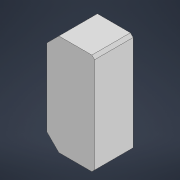
# Autodesk Inventor part: Carcasa
Saved by Autodesk Inventor 2022 (Build 260153000, 153)
## iProperties
Created: 2021-09-15
Part Number: Carcasa
Material: Generic
Document SubType Name: Sheet Metal
Designer: ARMU
Density: 1 g/cm^3
Sheet Metal Rule: Default
Appearance: Default
Author: ARMU
Autodesk Inventor part; units mm, degrees
ref_plane "YZ Plane" through (0, 0, 0) normal (1, 0, 0) x (0, 1, 0)
ref_plane "XZ Plane" through (0, 0, 0) normal (0, 1, 0) x (-1, 0, 0)
ref_plane "XY Plane" through (0, 0, 0) normal (0, 0, 1) x (1, 0, 0)
sketch "Sketch1" plane through (0, 0, 0) normal (0, 0, 1) x (1, 0, 0)
  line L0 (-272.7403, 778.9497) -> (12.2307, 778.9497)
  line L1 (12.2307, 778.9497) -> (35.7452, 755.4352)
  line L2 (35.7452, 755.4352) -> (35.7452, -69.5358)
  line L3 (35.7452, -69.5358) -> (12.2307, -93.0503)
  line L4 (12.2307, -93.0503) -> (-272.7403, -93.0503)
  line L5 (-376.2548, 10.4642) -> (-376.2548, 675.4352)
  line L6 (-376.2548, 675.4352) -> (-272.7403, 778.9497)
  line L7 (-376.2548, 10.4642) -> (-272.7403, -93.0503)
  circle A0 centre (35.7452, 778.9497) radius 23.5145 construction
  circle A1 centre (35.7452, -93.0503) radius 23.5145 construction
  circle A2 centre (-376.2548, 778.9497) radius 103.5145 construction
  circle A3 centre (-376.2548, -93.0503) radius 103.5145 construction
  line L8 (-271.4976, 775.9497) -> (-373.2548, 674.1926)
  line L9 (-373.2548, 674.1926) -> (-373.2548, 11.7068)
  line L10 (-373.2548, 11.7068) -> (-271.4976, -90.0503)
  line L11 (-271.4976, -90.0503) -> (10.9881, -90.0503)
  line L12 (10.9881, -90.0503) -> (32.7452, -68.2932)
  line L13 (32.7452, -68.2932) -> (32.7452, 754.1926)
  line L14 (32.7452, 754.1926) -> (10.9881, 775.9497)
  line L15 (10.9881, 775.9497) -> (-271.4976, 775.9497)
  line L16 (12.2307, -93.0503) -> (120.7988, -93.0503) construction
  line L17 (35.7452, -141.5714) -> (35.7452, 886.488) construction
  line L18 (124.1159, 778.9497) -> (-545.8501, 778.9497) construction
  line L19 (-376.2548, 913.6929) -> (-376.2548, -285.4862) construction
  line L20 (-520.4273, -93.0503) -> (301.4817, -93.0503) construction
  point P0 (0, 0)
  dimension "d2" = 47.029
  dimension "d0" = 872
  dimension "d1" = 412
  dimension "d3" = 47.029
  dimension "d4" = 207.029
  dimension "d5" = 207.029
  dimension "d6" = 3
  dimension "d7" = 3
  dimension "d8" = 3
  dimension "d9" = 3
  dimension "d10" = 3
  dimension "d11" = 3
  dimension "d12" = 3
  dimension "d13" = 3
  constraints: 42 end point, 12 point on line, 8 parallel, 6 point on circle, 4 vertical, 3 centre point, 3 horizontal, 2 collinear, 1 perpendicular, 1 vertical alignment, 2 other
  measures "d0" distance between parallel lines of L4 L0
  measures "d1" distance between parallel lines of L2 L5
  measures "d3" diameter of A1
  measures "d4" diameter of A2
  measures "d5" diameter of A3
  measures "d6" distance between parallel lines of L0 L15
  measures "d7" distance between parallel lines of L5 L9
  measures "d8" distance between parallel lines of L2 L13
  measures "d9" distance between parallel lines of L11 L4
  measures "d10" distance between parallel lines of L12 L3
  measures "d11" distance between parallel lines of L1 L14
  measures "d12" distance between parallel lines of L8 L6
  measures "d13" distance between parallel lines of L7 L10
extrude "Extrusion1" add sketch "Sketch1" along normal blind 330
sketch "Sketch2" plane through (0, 0, 330) normal (0, 0, 1) x (1, 0, 0)
  line L0 (-272.7403, 778.9497) -> (12.2307, 778.9497)
  line L1 (12.2307, 778.9497) -> (35.7452, 755.4352)
  line L2 (35.7452, 755.4352) -> (35.7452, -69.5358)
  line L3 (35.7452, -69.5358) -> (12.2307, -93.0503)
  line L4 (12.2307, -93.0503) -> (-272.7403, -93.0503)
  line L5 (-376.2548, 10.4642) -> (-376.2548, 675.4352)
  line L6 (-376.2548, 675.4352) -> (-272.7403, 778.9497)
  line L7 (-376.2548, 10.4642) -> (-272.7403, -93.0503)
  circle A0 centre (35.7452, 778.9497) radius 23.5145 construction
  circle A1 centre (35.7452, -93.0503) radius 23.5145 construction
  circle A2 centre (-376.2548, 778.9497) radius 103.5145 construction
  circle A3 centre (-376.2548, -93.0503) radius 103.5145 construction
  line L8 (12.2307, -93.0503) -> (120.7988, -93.0503) construction
  line L9 (35.7452, -141.5714) -> (35.7452, 886.488) construction
  line L10 (124.1159, 778.9497) -> (-545.8501, 778.9497) construction
  line L11 (-376.2548, 913.6929) -> (-376.2548, -285.4862) construction
  line L12 (-520.4273, -93.0503) -> (301.4817, -93.0503) construction
  point P0 (0, 0)
  point P1 (0, 0)
  dimension "d18" = 47.029
  dimension "d16" = 872
  dimension "d17" = 412
  dimension "d19" = 47.029
  dimension "d20" = 207.029
  dimension "d21" = 207.029
  constraints: 26 end point, 12 point on line, 6 point on circle, 4 vertical, 3 centre point, 3 horizontal, 2 collinear, 1 perpendicular, 1 vertical alignment, 2 other
  measures "d16" distance between parallel lines of L4 L0
  measures "d17" distance between parallel lines of L2 L5
  measures "d19" diameter of A1
  measures "d20" diameter of A2
  measures "d21" diameter of A3
extrude "Extrusion2" add sketch "Sketch2" along normal blind 3
equation "\"BendRadius\" = Thickness"
equation "\"BendReliefWidth\" = Thickness"
equation "\"BendReliefDepth\" = 0.5 * Thickness"
equation "\"CornerReliefSize\" = 4 * Thickness"
equation "\"MinimumRemnant\" = 2 * Thickness"
equation "\"TransitionRadius\" = BendRadius"
equation "\"JacobiRadiusSize\" = BendRadius"
equation "\"GapSize\" = Thickness"
equation "\"Thickness\" = 3.048"
body "Solid1"
